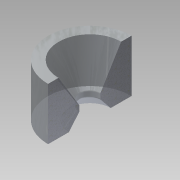
# Autodesk Inventor part: nozzle_small
Saved by Autodesk Inventor 2014 (Build 180170000, 170)
## iProperties
Created: 2013-10-01
Part Number: nozzle_small
Material: Glass
Document SubType Name: Modeling
Designer: Admin
Density: 1 g/cm^3
Appearance: Clear
Author: Admin
Autodesk Inventor part; units mm, degrees
ref_plane "YZ Plane" through (0, 0, 0) normal (1, 0, 0) x (0, 1, 0)
ref_plane "XZ Plane" through (0, 0, 0) normal (0, 1, 0) x (-1, 0, 0)
ref_plane "XY Plane" through (0, 0, 0) normal (0, 0, 1) x (1, 0, 0)
sketch "Sketch2" plane through (0, 0, 0) normal (0, 1, 0) x (-1, 0, 0)
  line L0 (4, 0) -> (4, 5)
  line L1 (0, -0.9936) -> (0, 4.4305)
  line L2 (4, 5) -> (4, 0)
  line L3 (1, 1.2185) -> (1, 1.7185)
  line L4 (1, 1.2185) -> (2, 0)
  line L5 (2, 0) -> (4, 0)
  line L6 (4, 5) -> (3, 5)
  line L7 (3, 5) -> (1, 1.7185)
  point P0 (0, 0)
  dimension "d4" = 5
  dimension "d16" = 1
  dimension "d18" = 2
  dimension "d24" = 1
  dimension "d25" = 4
  constraints: 16 end point, 2 parallel, 1 perpendicular
  measures "d4" distance of L0.start L0.end
  measures "d16" horizontal distance of L3.end point (0, 0)
  measures "d18" distance of point (0, 0) L4.end
  measures "d24" distance of L0.end L6.end
  measures "d25" distance of point (0, 0) L0.start
revolve "Revolution2" add sketch "Sketch2" angle 360 about axis through (0, 0, -0.9936) along (0, 0, 1)
fillet "Fillet3" radius 0.2 2 edges at (1, 0, 1.7185) (1, 0, 1.2185)
body "Solid2"
